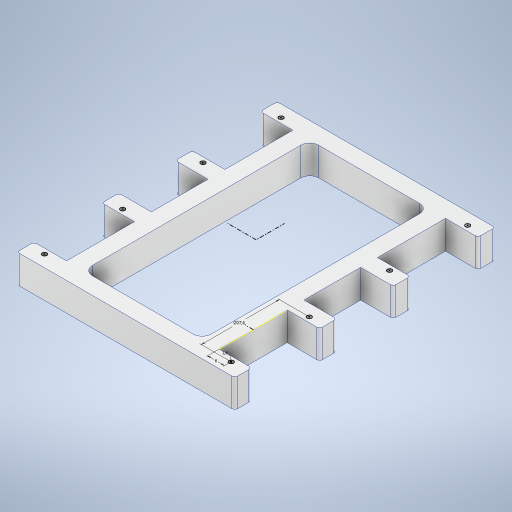
# Autodesk Inventor part: rapoukBasev4
Saved by Autodesk Inventor 2024 (Build 280153000, 153)
## iProperties
Created: 2023-06-17
Part Number: rapoukBasev4
Material: Aluminum 6061
Document SubType Name: Modeling
Designer: Roman
Density: 2.7 g/cm^3
Appearance: Aluminum - Flat
Description: Základní konstrukce
Mass: 59.5776 g
Surface Area: 124.22 cm^2
Volume: 22.0658 cm^3
Polotovar: KR...
Author: Roman
## iProperties of the stored document Basev1_3DPrint.ipt
Created: 2023-06-17
Part Number: Basev1_3DPrint
Material: Generic
Document SubType Name: Modeling
Designer: Roman
Density: 1 g/cm^3
Appearance: Default
Author: Roman
Autodesk Inventor part; units mm, degrees
ref_plane "YZ Plane" through (0, 0, 0) normal (1, 0, 0) x (0, 1, 0)
ref_plane "XZ Plane" through (0, 0, 0) normal (0, 1, 0) x (-1, 0, 0)
ref_plane "XY Plane" through (0, 0, 0) normal (0, 0, 1) x (1, 0, 0)
sketch "Sketch1" plane through (0, 0, 0) normal (0, 1, 0) x (-1, 0, 0)
  line L0 (38.5, 46) -> (38.5, -46)
  line L1 (38.5, -46) -> (-38.5, -46)
  line L2 (-38.5, -46) -> (-38.5, 46)
  line L3 (-38.5, 46) -> (38.5, -46) construction
  line L4 (38.5, 46) -> (-38.5, -46) construction
  line L5 (38.5, 46) -> (-38.5, 46)
  point P0 (0, 0)
  dimension "d0" = 77
  dimension "d1" = 92
  constraints: 12 end point, 2 midpoint, 1 horizontal, 1 parallel, 1 perpendicular
  measures "d0" distance of L0.end L1.end
  measures "d1" distance of L0.start L0.end
extrude "Extrusion1" add sketch "Sketch1" along normal blind 10
sketch "Sketch3" plane through (0, 10, 0) normal (0, 1, 0) x (1, 0, 0)
  line L0 (27, -46) -> (27, 46)
  line L1 (38.5, -46) -> (38.5, 46) projected
  line L2 (38.5, -40) -> (27, -40)
  line L3 (27, -40) -> (27, -16)
  line L4 (27, -16) -> (38.5, -16)
  line L5 (38.5, -16) -> (38.5, -40)
  line L6 (0, 0) -> (10, 0)
  line L7 (0, 0) -> (0, 10)
  line L8 (38.5, 40) -> (27, 40)
  line L9 (27, 16) -> (38.5, 16)
  line L10 (38.5, 16) -> (38.5, 40)
  line L11 (27, 40) -> (0, 40)
  line L12 (21, -34) -> (21, 40)
  line L13 (-27, -46) -> (-27, 46)
  line L14 (-38.5, -46) -> (-38.5, 46)
  line L15 (-38.5, -40) -> (-27, -40)
  line L16 (-27, -16) -> (-38.5, -16)
  line L17 (-38.5, 40) -> (-27, 40)
  line L18 (-27, 16) -> (-38.5, 16)
  line L19 (-27, 40) -> (0, 40)
  line L20 (-21, -34) -> (-21, 40)
  line L21 (27, 0) -> (38.5, 0)
  line L22 (38.5, 0) -> (38.5, -10)
  line L23 (38.5, -10) -> (27, -10)
  line L24 (27, -10) -> (27, 0)
  line L25 (38.5, 46) -> (38.5, -46)
  line L26 (38.5, 10) -> (27, 10)
  line L27 (-38.5, -10) -> (-27, -10)
  line L28 (-38.5, 10) -> (-27, 10)
  line L29 (-38.5, -46) -> (38.5, -46) projected
  line L30 (38.5, 46) -> (-38.5, 46) projected
  line L31 (-27, -40) -> (27, -40)
  line L32 (-21, -34) -> (-21, -40)
  line L33 (21, -34) -> (21, -40)
  line L34 (-32, -10) -> (-32, 10)
  point P0 (32.75, -40)
  point P1 (-27, -34)
  point P2 (27, 16)
  point P3 (38.5, 16)
  point P4 (38.5, 40)
  point P5 (27, 40)
  point P6 (38.5, -16)
  point P7 (27, -40)
  point P8 (-27, 40)
  point P9 (-38.5, 40)
  point P10 (-38.5, 16)
  point P11 (-38.5, -16)
  point P12 (-27, -40)
  point P13 (32.75, -16)
  point P14 (-38.5, 10)
  point P15 (-38.5, -10)
  point P16 (-27, -10)
  point P17 (27, -10)
  point P18 (38.5, 10)
  point P19 (27, 10)
  point P20 (-32.75, -40)
  point P21 (32.75, 0)
  point P22 (32.75, -10)
  dimension "d12" = 24
  dimension "d14" = 10
  dimension "d15" = 10
  dimension "d18" = 6
  dimension "d21" = 6
  dimension "d48" = 42
  dimension "d49" = 6
  dimension "d51" = 6
  dimension "d52" = 10
  dimension "d72" = 5
  constraints: 64 end point, 25 symmetric about line, 14 point on line, 7 perpendicular, 6 midpoint, 4 horizontal, 4 parallel, 2 vertical
  measures "d12" distance of L2.end L3.end
  measures "d14" distance of L6.start L6.end
  measures "d15" distance of L6.start L7.end
  measures "d18" distance between parallel lines of L12 L0
  measures "d21" distance from line of L23 point (32.75, -16)
  measures "d48" distance between parallel lines of L20 L12
  measures "d49" distance from line of point (-32.75, -40) L29
  measures "d51" distance between parallel lines of L30 L11
  measures "d52" distance of point (32.75, 0) point (32.75, -10)
  measures "d72" distance between parallel lines of L34 L13
extrude "Extrusion2" cut sketch "Sketch3" against normal through all contours L0 L4 L1 L2 | L31 L32 L20 L19 L11 L12 L33 | L15 L14 L16 L13 | L0 L21 L1 L23 | L0 L26 L1 L21 | L27 L34 L28 L13 | L8 L1 L9 L0 | L27 L14 L28 L34 | L13 L18 L14 L17
fillet "Fillet1" radius 3.175 4 edges at (21, 5, -40) (-21, 5, -40) (-21, 5, 40) (21, 5, 40)
fillet "Fillet2" radius 1 16 edges at (38.5, 5, 46) (38.5, 5, 40) (38.5, 5, 10) (38.5, 5, 16) (38.5, 5, -16) (38.5, 5, -10) (38.5, 5, -40) (38.5, 5, -46) (-38.5, 5, -46) (-38.5, 5, -40) (-38.5, 5, -16) (-38.5, 5, -10) (-38.5, 5, 10) (-38.5, 5, 16) (-38.5, 5, 40) (-38.5, 5, 46)
sketch "Sketch4" plane through (0, 10, 0) normal (0, 1, 0) x (1, 0, 0)
  line L0 (0, 0) -> (0, 10)
  line L1 (0, 0) -> (-10, 0)
  circle A0 centre (33, -41.8) radius 0.8
  line L2 (27, -40) -> (27, -16) projected
  line L3 (27, -28) -> (24, -28)
  circle A1 centre (33, -14.2) radius 0.8
  circle A2 centre (33, 41.8) radius 0.8
  circle A3 centre (33, 14.2) radius 0.8
  circle A4 centre (-33, -41.8) radius 0.8
  circle A5 centre (-33, -14.2) radius 0.8
  circle A6 centre (-33, 41.8) radius 0.8
  circle A7 centre (-33, 14.2) radius 0.8
  dimension "d27" = 1.6
  dimension "d29" = 27.6
  dimension "d30" = 6
  constraints: 8 centre point, 7 symmetric about line, 6 end point, 2 horizontal, 1 midpoint, 1 vertical, 7 other
  measures "d27" diameter of A0
  measures "d29" diameter of A0.centre L3
  measures "d30" horizontal distance of A0.centre L2.start
hole "Hole1" at (-33, 10, 41.8) at (-33, 10, 14.2) at (-33, 10, -14.2) at (-33, 10, -41.8) at (33, 10, -41.8) at (33, 10, -14.2) at (33, 10, 14.2) at (33, 10, 41.8) direction (0, -1, 0) diameter 1.567 depth 10 thread size "M2x0.4" class "6H" standard "ISO Metric profile"
body "Solid1"
